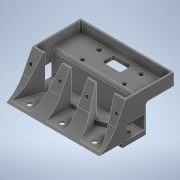
# Autodesk Inventor part: Corpo
Saved by Autodesk Inventor 2021 (Build 250183000, 183)
## iProperties
Created: 2022-11-17
Part Number: Corpo
Material: Plástico PC/ABS
Document SubType Name: Modeling
Designer: nicho
Density: 0.357273 g/cm^3
Appearance: Liso - Preto
Mass: 16.6236 g
Surface Area: 359.302 cm^2
Volume: 46.5292 cm^3
Author: nicho
Autodesk Inventor part; units mm, degrees
ref_plane "YZ Plane" through (0, 0, 0) normal (1, 0, 0) x (0, 1, 0)
ref_plane "XZ Plane" through (0, 0, 0) normal (0, 1, 0) x (-1, 0, 0)
ref_plane "XY Plane" through (0, 0, 0) normal (0, 0, 1) x (1, 0, 0)
sketch "Esboço1" plane through (0, 0, 0) normal (1, 0, 0) x (0, 1, 0)
  line L0 (-19.25, -25) -> (19.25, -25)
  line L1 (19.25, -25) -> (19.25, 25)
  line L2 (19.25, 25) -> (-19.25, 25)
  line L3 (-19.25, 25) -> (-19.25, -25)
  line L4 (-19.25, -25) -> (19.25, 25) construction
  line L5 (19.25, -25) -> (-19.25, 25) construction
  point P0 (0, 0)
  dimension "d0" = 38.5
  dimension "d1" = 50
  constraints: 12 end point, 2 midpoint, 2 parallel, 1 horizontal, 1 perpendicular
  measures "d0" distance of L2.end L1.end
  measures "d1" distance of L1.end L0.end
extrude "Extrusão1" add sketch "Esboço1" along normal mid plane 100
sketch "Esboço2" plane through (50, 0, 0) normal (1, 0, 0) x (0, 0, -1)
  line L0 (25, 19.25) -> (-25, 19.25) projected
  line L1 (25, 19.25) -> (23.5, 19.25)
  line L2 (23.5, 19.25) -> (3, 19.25)
  line L3 (-25, 19.25) -> (-25, -19.25) construction
  line L4 (-25, -19.25) -> (-40.6046, -27.5471) construction
  line L5 (-40.6046, -27.5471) -> (0.8044, -27.5471) construction
  circle A0 centre (-44.3905, 17.2183) radius 41.3029
  line L6 (-7.5894, -1.5328) -> (3, 19.25)
  line L7 (25, 19.25) -> (-25, 19.25) projected
  line L8 (-25, 19.25) -> (-25, -19.25) projected
  line L9 (-25, -19.25) -> (25, -19.25) projected
  line L10 (25, -19.25) -> (25, 19.25) projected
  point P0 (0, 0)
  dimension "d4" = 1.5
  dimension "d5" = 20.5
  dimension "d6" = 28
  dimension "d7" = 63
  constraints: 10 end point, 2 point on circle, 2 point on line, 2 tangent, 1 centre point, 1 perpendicular
  measures "d4" distance of L0.start L1.end
  measures "d5" distance of L1.end L2.end
  measures "d6" angle of L5 L4
  measures "d7" angle of L5 L6
extrude "Extrusão2" cut sketch "Esboço2" against normal through all contours L6 A0 L0 | L8 L0 A0 picked at (-22.6753, -4.8585)
sketch "Esboço3" plane through (-50, 19.25, -25) normal (0, 1, 0) x (1, 0, 0)
  line L0 (0, -22) -> (100, -22) projected
  line L1 (100, 0) -> (100, -22) projected
  line L2 (100, 0) -> (0, 0) projected
  line L3 (0, -22) -> (0, 0) projected
  line L4 (1.5, -1.5) -> (98.5, -1.5)
  line L5 (98.5, -1.5) -> (98.5, -20.5)
  line L6 (98.5, -20.5) -> (1.5, -20.5)
  line L7 (1.5, -20.5) -> (1.5, -1.5)
  point P0 (98.5, -22)
  point P1 (1.5, -22)
  dimension "d14" = 1.5
  constraints: 8 end point, 2 point on line, 3 other
  measures "d14" distance between parallel lines of L2 L4
extrude "Extrusão3" cut sketch "Esboço3" against normal blind 37 contours L4 L5 L6 L7
ref_plane "Plano de trabalho1" through (-48.5, -17.75, -23.5) normal (0, 1, 0) x (1, 0, 0)
sketch "Esboço4" plane through (-48.5, -17.75, -23.5) normal (0, 1, 0) x (1, 0, 0)
  line L0 (39, -19) -> (58, -19)
  line L1 (58, -19) -> (58, -109.0722)
  line L2 (58, -109.0722) -> (39, -109.0722)
  line L3 (39, -109.0722) -> (39, -19)
  line L4 (39, -19) -> (58, -109.0722) construction
  line L5 (58, -19) -> (39, -109.0722) construction
  line L6 (97, -19) -> (0, -19) projected
  line L7 (-1.5, -20.5) -> (-1.5, 1.5) projected
  line L8 (10.7728, -19) -> (28.62, -25.5174)
  line L9 (28.62, -25.5174) -> (-1.8924, -109.0722)
  line L10 (-1.8924, -109.0722) -> (-19.7396, -102.5548)
  line L11 (-19.7396, -102.5548) -> (10.7728, -19)
  line L12 (-1.5, -48.5) -> (98.5, -48.5) projected
  line L13 (-1.5, -48.5) -> (-1.5, -31.0894) projected
  line L14 (48.5, -64.0361) -> (48.5, 0)
  line L15 (0, 0) -> (97, 0) projected
  line L16 (86.2272, -19) -> (68.38, -25.5174)
  line L17 (68.38, -25.5174) -> (98.8924, -109.0722)
  line L18 (98.8924, -109.0722) -> (116.7396, -102.5548)
  line L19 (116.7396, -102.5548) -> (86.2272, -19)
  line L20 (-1.5, -31.0894) -> (-1.5, -20.5) projected
  line L21 (98.5, -31.0894) -> (-1.5, -31.0894) projected
  line L22 (98.5, -20.5) -> (98.5, -31.0894) projected
  line L23 (-1.5, -20.5) -> (98.5, -20.5) projected
  line L24 (-1.5, -48.5) -> (-1.5, -31.0894) projected
  line L25 (-1.5, -48.5) -> (98.5, -48.5) projected
  line L26 (98.5, -31.0894) -> (98.5, -48.5) projected
  line L27 (98.5, -31.0894) -> (-1.5, -31.0894) projected
  line L28 (97, 0) -> (97, -19) projected
  line L29 (97, -19) -> (0, -19) projected
  line L30 (0, -19) -> (0, 0) projected
  line L31 (0, 0) -> (97, 0) projected
  line L32 (-1.5, -20.5) -> (98.5, -20.5) projected
  line L33 (98.5, 1.5) -> (98.5, -20.5) projected
  line L34 (98.5, 1.5) -> (-1.5, 1.5) projected
  line L35 (-1.5, -20.5) -> (-1.5, 1.5) projected
  line L36 (28.62, -25.5174) -> (31, -19)
  line L37 (97, -19) -> (0, -19) projected
  line L38 (68.38, -25.5174) -> (66, -19)
  point P0 (48.5, -23.5)
  point P1 (0, -48.5)
  point P2 (86.2272, -19)
  dimension "d15" = 19
  dimension "d16" = 50
  dimension "d17" = 19
  dimension "d19" = 1.5
  dimension "d90" = 8
  constraints: 34 end point, 5 point on line, 4 parallel, 4 symmetric about line, 3 midpoint, 2 collinear, 2 perpendicular, 1 horizontal, 1 horizontal alignment, 2 other
  measures "d15" distance of L1.end L2.end
  measures "d16" distance from line of L7 L14.start
  measures "d17" distance between parallel lines of L9 L11
  measures "d19" distance from line of L13 point (0, -48.5)
  measures "d90" distance from line of L3 L36.end
extrude "Extrusão4" cut sketch "Esboço4" along normal through all contours L0 L14 L23 L3 | L0 L1 L23 L14 | L23 L14 L21 L3 | L36 L23 L8 L6 | L23 L1 L21 L14 | L21 L14 L12 L3 | L36 L8 L23 | L8 L23 L11 | L6 L16 L23 L38 | L21 L1 L12 L14 | L12 L1 L2 L3 | L21 L11 L23 L8 L9 | L9 L12 L11 L21 | L23 L16 L38 | L19 L23 L16 | L9 L10 L11 L12 | L21 L19 L12 L17 | L17 L16 L23 L19 L21 | L12 L19 L18 L17
sketch "Esboço8" plane through (-50, -19.25, -25) normal (0, -1, 0) x (1, 0, 0)
  line L0 (100, 50) -> (100, 0) projected
  line L1 (0, 0) -> (0, 50) projected
  line L2 (100, 0) -> (0, 0)
  line L3 (0, 0) -> (0, 25)
  line L4 (0, 25) -> (100, 25)
  line L5 (100, 25) -> (100, 0)
  point P0 (50, 25)
  dimension "d32" = 25
  constraints: 8 end point, 2 parallel, 1 horizontal, 1 midpoint, 1 perpendicular
  measures "d32" distance of L2.end L3.end
extrude "Extrusão7" add sketch "Esboço8" along normal blind 4.85
sketch "Esboço10" plane through (-50, -17.75, -25) normal (0, 1, 0) x (1, 0, 0)
  line L0 (40.5, -20.5) -> (32.5, -20.5) projected
  line L1 (12.2728, -20.5) -> (32.5, -20.5)
  line L2 (40.5, -20.5) -> (59.5, -20.5)
  line L3 (67.5, -20.5) -> (59.5, -20.5) projected
  line L4 (98.5, -20.5) -> (87.7272, -20.5) projected
  line L5 (67.5, -20.5) -> (87.7272, -20.5)
  line L6 (7.858, -32.5894) -> (11.725, -22) projected
  line L7 (98.5, -20.5) -> (87.7272, -20.5) projected
  line L8 (98.5, -1.5) -> (98.5, -20.5) projected
  line L9 (1.5, -1.5) -> (98.5, -1.5) projected
  line L10 (1.5, -20.5) -> (1.5, -1.5) projected
  line L11 (12.2728, -20.5) -> (1.5, -20.5) projected
  line L12 (12.2728, -20.5) -> (2.4458, -47.4099) projected
  line L13 (22.6731, -47.4099) -> (2.4458, -47.4099) projected
  line L14 (22.6731, -47.4099) -> (32.5, -20.5) projected
  line L15 (40.5, -20.5) -> (32.5, -20.5) projected
  line L16 (40.5, -20.5) -> (40.5, -47.4099) projected
  line L17 (59.5, -47.4099) -> (40.5, -47.4099) projected
  line L18 (59.5, -47.4099) -> (59.5, -20.5) projected
  line L19 (67.5, -20.5) -> (59.5, -20.5) projected
  line L20 (67.5, -20.5) -> (77.3269, -47.4099) projected
  line L21 (97.5542, -47.4099) -> (77.3269, -47.4099) projected
  line L22 (97.5542, -47.4099) -> (87.7272, -20.5) projected
  line L23 (31.9522, -22) -> (28.0852, -32.5894) projected
  line L24 (88.275, -22) -> (100, -22) projected
  line L25 (0, -25) -> (100, -25) projected
  line L26 (40.5, -20.5) -> (40.5, -47.4099) projected
  line L27 (59.5, -22) -> (59.5, -32.5894) projected
  line L28 (71.9148, -32.5894) -> (68.0478, -22) projected
  line L29 (88.275, -22) -> (92.142, -32.5894) projected
  line L30 (12.2728, -20.5) -> (2.4458, -47.4099) projected
  line L31 (22.6731, -47.4099) -> (32.5, -20.5) projected
  line L32 (31.9522, -22) -> (40.5, -22) projected
  line L33 (40.5, -22) -> (59.5, -22)
  line L34 (69.1433, -25) -> (77.3585, -22)
  line L35 (0, -22) -> (11.725, -22) projected
  line L36 (21.1494, -21.4551) -> (30.8567, -25)
  line L37 (21.1494, -21.4551) -> (21.1494, -20.5)
  line L38 (77.3585, -22) -> (77.3585, -20.5)
  point P0 (50, -25)
  constraints: 16 end point, 7 point on line, 4 horizontal, 4 perpendicular, 1 horizontal alignment
extrude "Extrusão9" add sketch "Esboço10" along normal blind 5 contours L2 L18 L33 L16 | L14 L36 L37 L1 | L5 L38 L34 L20
sketch "Esboço11" plane through (-50, -17.75, -25) normal (0, 1, 0) x (1, 0, 0)
  line L0 (98.5, -20.5) -> (87.7272, -20.5) projected
  line L1 (98.5, -1.5) -> (98.5, -20.5) projected
  line L2 (1.5, -1.5) -> (98.5, -1.5) projected
  line L3 (1.5, -20.5) -> (1.5, -1.5) projected
  line L4 (12.2728, -20.5) -> (1.5, -20.5) projected
  line L5 (12.2728, -20.5) -> (2.4458, -47.4099) projected
  line L6 (22.6731, -47.4099) -> (2.4458, -47.4099) projected
  line L7 (22.6731, -47.4099) -> (30.8567, -25) projected
  line L8 (77.3585, -20.5) -> (21.1494, -20.5) projected
  line L9 (77.3585, -20.5) -> (77.3585, -22) projected
  line L10 (77.3585, -22) -> (69.1433, -25) projected
  line L11 (69.1433, -25) -> (77.3269, -47.4099) projected
  line L12 (97.5542, -47.4099) -> (77.3269, -47.4099) projected
  line L13 (97.5542, -47.4099) -> (87.7272, -20.5) projected
  line L14 (30.8567, -25) -> (21.1494, -21.4551) projected
  line L15 (21.1494, -21.4551) -> (21.1494, -20.5) projected
  line L16 (98.5, -20.5) -> (87.7272, -20.5) projected
  line L17 (12.2728, -20.5) -> (87.7272, -20.5)
  point P0 (50, -25)
  point P1 (21.1494, -20.5)
  constraints: 2 end point, 1 horizontal
extrude "Extrusão10" cut sketch "Esboço11" against normal blind 4.85 contours L0 L17 L8 L4 L3 L2 L1
sketch "Esboço12" plane through (-50, 0, 0) normal (-1, 0, 0) x (0, 0, 1)
  line L0 (-23.5, -19.1) -> (-4.5, -19.1)
  line L1 (-4.5, -19.1) -> (-4.5, -4.1)
  line L2 (-4.5, -4.1) -> (-23.5, -4.1)
  line L3 (-23.5, -4.1) -> (-23.5, -19.1)
  line L4 (-25, 19.25) -> (-25, -24.1) projected
  line L5 (0, -24.1) -> (-25, -24.1) projected
  point P0 (0, 0)
  dimension "d41" = 19
  dimension "d42" = 15
  dimension "d43" = 1.5
  dimension "d44" = 5
  constraints: 8 end point, 2 parallel, 1 horizontal, 1 perpendicular
  measures "d41" distance of L2.end L1.end
  measures "d42" distance of L1.end L0.end
  measures "d43" distance between parallel lines of L4 L3
  measures "d44" distance between parallel lines of L5 L0
extrude "Extrusão11" cut sketch "Esboço12" against normal through all
sketch "Esboço13" plane through (-50, -22.6, -25) normal (0, 1, 0) x (1, 0, 0)
  line L0 (1.5, -1.5) -> (98.5, -1.5) projected
  line L1 (98.5, -20.5) -> (1.5, -20.5) projected
  line L2 (1.5, -1.5) -> (16, -1.5)
  line L3 (16, -1.5) -> (16, -20.5)
  line L4 (16, -20.5) -> (1.5, -20.5)
  line L5 (1.5, -20.5) -> (1.5, -1.5)
  line L6 (98.5, -20.5) -> (98.5, -1.5) projected
  line L7 (59.5, -20.5) -> (67.5, -20.5) projected
  line L8 (98.5, -1.5) -> (84, -1.5)
  line L9 (84, -1.5) -> (84, -20.5)
  line L10 (84, -20.5) -> (98.5, -20.5)
  line L11 (98.5, -20.5) -> (98.5, -1.5)
  point P0 (50, -25)
  point P1 (87.7272, -20.5)
  point P2 (84, -1.5)
  dimension "d47" = 14.5
  dimension "d48" = 14.5
  constraints: 16 end point, 4 parallel, 2 perpendicular, 2 point on line, 1 horizontal
  measures "d47" distance of L3.end L4.end
  measures "d48" distance of L10.end L9.end
extrude "Extrusão12" add sketch "Esboço13" along normal up to surface (3.5 mm away) contours L0 L3 L1 L5 | L0 L6 L1 L9
sketch "Esboço14" plane through (-50, -19.1, -4.5) normal (0, 1, 0) x (1, 0, 0)
  line L0 (16, 19) -> (16, 0) projected
  line L1 (100, 0) -> (0, 0) projected
  line L2 (16, 19) -> (14.5, 19)
  line L3 (14.5, 19) -> (14.5, 0)
  line L4 (14.5, 0) -> (16, 0)
  line L5 (16, 0) -> (16, 19)
  line L6 (84, 19) -> (100, 19) projected
  line L7 (59.5, 0) -> (67.5, 0) projected
  line L8 (84, 19) -> (85.5, 19)
  line L9 (85.5, 19) -> (85.5, 0)
  line L10 (85.5, 0) -> (84, 0)
  line L11 (84, 0) -> (84, 19)
  point P0 (50, -4.5)
  point P1 (87.7272, 0)
  point P2 (84, 0)
  dimension "d51" = 1.5
  dimension "d52" = 1.5
  constraints: 16 end point, 4 parallel, 2 horizontal, 2 perpendicular, 2 point on line
  measures "d51" distance of L4.end L3.end
  measures "d52" distance of L9.end L10.end
extrude "Extrusão13" add sketch "Esboço14" along normal up to surface (6.35 mm away)
sketch "Esboço15" plane through (50, 19.25, -25) normal (0, 0, -1) x (-1, 0, 0)
  line L0 (0, 0) -> (0, -20.7828) projected
  line L1 (100, 0) -> (100, -43.35) projected
  line L2 (0, 0) -> (100, 0)
  line L3 (100, 0) -> (100, -13)
  line L4 (100, -13) -> (0, -13)
  line L5 (0, -13) -> (0, 0)
  point P0 (50, -19.25)
  point P1 (0, -13)
  dimension "d55" = 13
  constraints: 8 end point, 2 parallel, 1 horizontal, 1 perpendicular, 1 point on line
  measures "d55" distance between parallel lines of L2 L4
extrude "Extrusão14" add sketch "Esboço15" along normal blind 30
sketch "Esboço16" plane through (-50, 6.25, -25) normal (0, -1, 0) x (1, 0, 0)
  line L0 (77.5, -30) -> (22.5, -30)
  line L1 (22.5, -30) -> (22.5, 0)
  line L2 (22.5, 0) -> (77.5, 0)
  line L3 (77.5, 0) -> (77.5, -30)
  line L4 (77.5, -30) -> (22.5, 0) construction
  line L5 (22.5, -30) -> (77.5, 0) construction
  line L6 (0, 0) -> (100, 0) projected
  line L7 (100, -30) -> (0, -30) projected
  line L8 (0, 0) -> (0, -30) projected
  point P0 (50, 25)
  point P1 (50, -15)
  dimension "d58" = 55
  dimension "d59" = 50
  constraints: 12 end point, 2 midpoint, 2 parallel, 2 point on line, 1 horizontal, 1 perpendicular
  measures "d58" distance of L1.end L2.end
  measures "d59" distance from line of L8 point (50, -15)
extrude "Extrusão15" add sketch "Esboço16" along normal blind 2.85 contours L0 L1 L2 L3
sketch "Esboço17" plane through (-48.5, 19.25, -23.5) normal (0, 1, 0) x (1, 0, 0)
  line L0 (97, 0) -> (97, -19) projected
  line L1 (97, 0) -> (0, 0)
  line L2 (0, 0) -> (0, 30)
  line L3 (0, 30) -> (97, 30)
  line L4 (97, 30) -> (97, 0)
  line L5 (86.2272, -19) -> (86.775, -20.5) projected
  line L6 (86.775, -20.5) -> (98.5, -20.5) projected
  line L7 (98.5, -20.5) -> (98.5, 31.5) projected
  line L8 (-1.5, 31.5) -> (98.5, 31.5) projected
  line L9 (-1.5, -20.5) -> (-1.5, 31.5) projected
  line L10 (-1.5, -20.5) -> (10.225, -20.5) projected
  line L11 (10.225, -20.5) -> (10.7728, -19) projected
  line L12 (10.7728, -19) -> (0, -19) projected
  line L13 (0, -19) -> (0, 0) projected
  line L14 (0, 0) -> (97, 0) projected
  line L15 (97, 0) -> (97, -19) projected
  line L16 (97, -19) -> (86.2272, -19) projected
  point P0 (48.5, -23.5)
  dimension "d62" = 1.5
  constraints: 8 end point, 2 parallel, 1 horizontal, 1 perpendicular, 1 point on line
  measures "d62" distance between parallel lines of L8 L3
extrude "Extrusão16" cut sketch "Esboço17" against normal blind 11.5 contours L1 L2 L3 L4
fillet "Arredondamento2" radius 2.85 3 edges at (0, 7.75, -23.5) (38.75, 6.25, -25) (-38.75, 6.25, -25)
fillet "Arredondamento3" radius 1.5 4 edges at (-48.5, 13.5, -53.5) (48.5, 13.5, -53.5) (48.5, 7.575, -4.5) (-48.5, 7.575, -4.5)
sketch "Esboço18" plane through (-50, 3.4, -25) normal (0, -1, 0) x (1, 0, 0)
  line L0 (0, 0) -> (100, 0) projected
  line L1 (77.5, -30) -> (77.5, 0) projected
  line L2 (22.5, 0) -> (22.5, -30) projected
  line L3 (22.5, -30) -> (77.5, -30) projected
  point P0 (50, 25)
  point P1 (72.5, -22.5)
  point P2 (27.5, -22.5)
  point P3 (27.5, -4.5)
  point P4 (72.5, -4.5)
  dimension "d69" = 4.5
  dimension "d70" = 5
  dimension "d71" = 5
  dimension "d72" = 7.5
  constraints: 2 horizontal alignment, 2 vertical alignment
  measures "d69" distance from line of L0 point (72.5, -4.5)
  measures "d70" distance from line of L1 point (72.5, -4.5)
  measures "d71" distance from line of L2 point (27.5, -4.5)
  measures "d72" distance from line of L3 point (72.5, -22.5)
hole "Furo1" at (22.5, 3.4, -47.5) at (-22.5, 3.4, -47.5) at (-22.5, 3.4, -29.5) at (22.5, 3.4, -29.5) direction (0, 1, 0) diameter 4 end through all start extended yes
chamfer "Chanfro1" distance 1 angle 45 4 edges at (-22.5, 7.75, -45.5) (-22.5, 7.75, -27.5) (22.5, 7.75, -27.5) (22.5, 7.75, -45.5)
sketch "Esboço19" plane through (-48.5, 7.75, -23.5) normal (0, 1, 0) x (1, 0, 0)
  line L0 (38.5, 26.5) -> (58.5, 26.5)
  line L1 (58.5, 26.5) -> (58.5, 14)
  line L2 (58.5, 14) -> (38.5, 14)
  line L3 (38.5, 14) -> (38.5, 26.5)
  line L4 (38.5, 26.5) -> (58.5, 14) construction
  line L5 (58.5, 26.5) -> (38.5, 14) construction
  line L6 (-1.5, -20.5) -> (-1.5, 31.5) projected
  line L7 (-1.5, 31.5) -> (98.5, 31.5) projected
  point P0 (48.5, -23.5)
  point P1 (48.5, 20.25)
  dimension "d83" = 20
  dimension "d84" = 12.5
  dimension "d85" = 50
  dimension "d86" = 5
  constraints: 12 end point, 2 midpoint, 2 parallel, 1 horizontal, 1 perpendicular
  measures "d83" distance of L1.end L2.end
  measures "d84" distance of L0.end L1.end
  measures "d85" distance from line of L6 point (48.5, 20.25)
  measures "d86" distance between parallel lines of L7 L0
extrude "Extrusão17" cut sketch "Esboço19" against normal through all
fillet "Arredondamento5" radius 2 4 edges at (-10, 5.575, -37.5) (10, 5.575, -37.5) (-10, 5.575, -50) (10, 5.575, -50)
sketch "Esboço20" plane through (-50, -17.75, -25) normal (0, 1, 0) x (1, 0, 0)
  line L0 (0, -22) -> (0, 30) projected
  line L1 (0, -50) -> (100, -50) projected
  line L2 (2.4458, -47.4099) -> (7.858, -32.5894) projected
  line L3 (92.142, -32.5894) -> (97.5542, -47.4099) projected
  point P0 (50, -25)
  point P1 (50, -40)
  point P2 (15, -40)
  point P3 (85, -40)
  dimension "d91" = 50
  dimension "d92" = 10
  dimension "d120" = 35
  dimension "d121" = 35
  constraints: 2 horizontal alignment
  measures "d91" distance from line of L0 point (50, -40)
  measures "d92" distance from line of L1 point (50, -40)
  measures "d120" distance of point (15, -40) point (50, -40)
  measures "d121" distance of point (85, -40) point (50, -40)
hole "Furo2" at (0, -17.75, 15) at (-35, -17.75, 15) at (35, -17.75, 15) direction (0, -1, 0) diameter 4 end through all start extended yes countersink diameter 6 countersink angle 90
sketch "Esboço21" plane through (-50, -19.1, -4.5) normal (0, 1, 0) x (1, 0, 0)
  line L0 (0, -1.5) -> (0, 50.5) projected
  line L1 (100, -1.5) -> (100, 50.5) projected
  line L2 (12.2728, 0) -> (3, 0) projected
  circle A0 centre (50, -19.5) radius 2 projected
  point P0 (50, -4.5)
  point P1 (7, 9.5)
  point P2 (93, 9.5)
  dimension "d126" = 29
  dimension "d127" = 43
  dimension "d128" = 43
  constraints: 1 horizontal alignment
  measures "d126" vertical distance of A0.centre point (7, 9.5)
  measures "d127" horizontal distance of A0.centre point (7, 9.5)
  measures "d128" horizontal distance of point (93, 9.5) A0.centre
hole "Furo3" at (-43, -19.1, -14) at (43, -19.1, -14) direction (0, -1, 0) diameter 4 end through all start extended yes countersink diameter 6 countersink angle 90
sketch "Esboço22" plane through (-50, -22.6, -25) normal (0, 1, 0) x (1, 0, 0)
  circle A0 centre (7, -11) radius 3 projected
  line L0 (14.5, -20.5) -> (14.5, -1.5) projected
  line L1 (0, -1.5) -> (14.5, -1.5) projected
  line L2 (0, -20.5) -> (0, -1.5) projected
  line L3 (14.5, -20.5) -> (0, -20.5) projected
  circle A1 centre (50, -40) radius 3 projected
  line L4 (59.5, -25) -> (40.5, -25) projected
  line L5 (40.5, -25) -> (40.5, -47.4099) projected
  line L6 (59.5, -47.4099) -> (40.5, -47.4099) projected
  line L7 (59.5, -47.4099) -> (59.5, -25) projected
  line L8 (85.5, -1.5) -> (85.5, -20.5) projected
  line L9 (100, -1.5) -> (100, -20.5) projected
  line L10 (85.5, -1.5) -> (100, -1.5) projected
  line L11 (100, -20.5) -> (85.5, -20.5) projected
  point P0 (50, -25)
  point P1 (50, -11)
  constraints: 1 horizontal alignment, 1 vertical alignment
hole "Furo4" at (0, -22.6, -14) direction (0, -1, 0) diameter 4 end through all start extended yes countersink diameter 6 countersink angle 90
ref_plane "Plano de trabalho2" through (-9.5, 19.25, -3) normal (0, 0.4539905, 0.8910065) x (1, 0, 0)
sketch "Esboço23" plane through (-9.5, 19.25, -3) normal (0, 0.4539905, 0.8910065) x (1, 0, 0)
  line L0 (0, -23.3251) -> (0, 0) projected
  line L1 (-8.5478, 0) -> (0, 0) projected
  line L2 (-8.5478, 0) -> (-12.4148, -23.3251) projected
  line L3 (0, -23.3251) -> (-12.4148, -23.3251) projected
  line L4 (31.4148, -23.3251) -> (27.5478, 0) projected
  line L5 (19, 0) -> (27.5478, 0) projected
  line L6 (19, 0) -> (19, -23.3251) projected
  line L7 (31.4148, -23.3251) -> (19, -23.3251) projected
  line L8 (47.775, 0) -> (51.642, -23.3251) projected
  line L9 (59.5, -23.3251) -> (51.642, -23.3251) projected
  line L10 (59.5, 0) -> (59.5, -23.3251) projected
  line L11 (47.775, 0) -> (59.5, 0) projected
  line L12 (-32.642, -23.3251) -> (-28.775, 0) projected
  line L13 (-40.5, 0) -> (-28.775, 0) projected
  line L14 (-40.5, -23.3251) -> (-40.5, 0) projected
  line L15 (-32.642, -23.3251) -> (-40.5, -23.3251) projected
  point P0 (9.5, -18.5138)
  point P1 (-5, -13.3251)
  point P2 (-36.5, -13.3251)
  point P3 (24, -13.3251)
  point P4 (55.5, -13.3251)
  dimension "d129" = 4
  dimension "d130" = 4
  dimension "d131" = 5
  dimension "d132" = 5
  dimension "d133" = 10
  constraints: 3 horizontal alignment
  measures "d129" distance from line of L10 point (55.5, -13.325)
  measures "d130" distance from line of L14 point (-36.5, -13.325)
  measures "d131" distance from line of L0 point (-5, -13.325)
  measures "d132" distance from line of L6 point (24, -13.325)
  measures "d133" distance from line of L7 point (24, -13.325)
hole "Furo5" at (-14.5, 7.3772, 3.0495) at (-46, 7.3772, 3.0495) at (14.5, 7.3772, 3.0495) at (46, 7.3772, 3.0495) direction (0, -0.4539905, -0.8910065) diameter 4 depth 5 start extended yes
sketch "Esboço24" plane through (-50, -17.75, -25) normal (0, 1, 0) x (1, 0, 0)
  circle A0 centre (15, -40) radius 3 projected
  line L0 (87.7272, -20.5) -> (85.5, -20.5) projected
  line L1 (16, -20.5) -> (14.5, -20.5) projected
  line L2 (14.5, -20.5) -> (12.2728, -20.5) projected
  line L3 (12.2728, -20.5) -> (2.4458, -47.4099) projected
  line L4 (22.6731, -47.4099) -> (2.4458, -47.4099) projected
  line L5 (22.6731, -47.4099) -> (30.8567, -25) projected
  line L6 (30.8567, -25) -> (21.1494, -21.4551) projected
  line L7 (21.1494, -21.4551) -> (21.1494, -20.5) projected
  circle A1 centre (85, -40) radius 3 projected
  line L8 (87.7272, -20.5) -> (85.5, -20.5) projected
  line L9 (85.5, -20.5) -> (84, -20.5) projected
  line L10 (84, -20.5) -> (77.3585, -20.5) projected
  line L11 (77.3585, -20.5) -> (77.3585, -22) projected
  line L12 (77.3585, -22) -> (69.1433, -25) projected
  line L13 (69.1433, -25) -> (77.3269, -47.4099) projected
  line L14 (97.5542, -47.4099) -> (77.3269, -47.4099) projected
  line L15 (97.5542, -47.4099) -> (87.7272, -20.5) projected
  line L16 (21.1494, -21.4551) -> (30.8567, -25) projected
  line L17 (21.1494, -21.4551) -> (16, -19.5747)
  line L18 (77.3585, -22) -> (84, -19.5747)
  line L19 (69.1433, -25) -> (77.3585, -22) projected
  line L20 (32.5, -20.5) -> (21.1494, -20.5) projected
  line L21 (21.1494, -20.5) -> (16, -18.6196)
  line L22 (16, -1.5) -> (16, -20.5) projected
  line L23 (77.3585, -22) -> (77.3585, -20.5) projected
  line L24 (77.3585, -20.5) -> (84, -18.0747)
  line L25 (84, -20.5) -> (84, -1.5) projected
  line L26 (21.1494, -20.5) -> (16, -20.5) projected
  line L27 (16, -20.5) -> (14.5, -20.5) projected
  line L28 (14.5, -20.5) -> (12.2728, -20.5) projected
  line L29 (12.2728, -20.5) -> (2.4458, -47.4099) projected
  line L30 (22.6731, -47.4099) -> (2.4458, -47.4099) projected
  line L31 (22.6731, -47.4099) -> (30.8567, -25) projected
  line L32 (30.8567, -25) -> (21.1494, -21.4551) projected
  line L33 (21.1494, -21.4551) -> (21.1494, -20.5) projected
  line L34 (85.5, -20.5) -> (84, -20.5) projected
  line L35 (84, -20.5) -> (77.3585, -20.5) projected
  line L36 (77.3585, -20.5) -> (77.3585, -22) projected
  line L37 (77.3585, -22) -> (69.1433, -25) projected
  line L38 (69.1433, -25) -> (77.3269, -47.4099) projected
  line L39 (97.5542, -47.4099) -> (77.3269, -47.4099) projected
  line L40 (97.5542, -47.4099) -> (87.7272, -20.5) projected
  line L41 (21.1494, -20.5) -> (16, -20.5) projected
  point P0 (50, -25)
  point P1 (16, -17.5)
  point P2 (84, -17.5)
  point P3 (16, -4.5)
  point P4 (84, -4.5)
  point P5 (81.466, -20.5)
  point P6 (18.534, -20.5)
  constraints: 8 end point, 2 collinear, 2 parallel, 2 point on line
extrude "Extrusão18" add sketch "Esboço24" along normal mid plane 10 contours L10 L18 L25 | L18 L11 L10 | L10 L24 L25 L18 | L22 L17 L26 | L22 L21 L26 L17 | L26 L7 L17
sketch "Esboço26" plane through (-50, -12.75, -25) normal (0, 1, 0) x (1, 0, 0)
  line L0 (18.534, -20.5) -> (30.8567, -25) projected
  line L1 (18.534, -20.5) -> (14.5, -19.0269)
  line L2 (14.5, -20.5) -> (14.5, -1.5) projected
  line L3 (21.1494, -20.5) -> (16, -18.6196) projected
  line L4 (18.534, -20.5) -> (30.8567, -25) projected
  line L5 (32.5, -20.5) -> (30.8567, -25) projected
  line L6 (32.5, -20.5) -> (21.1494, -20.5) projected
  line L7 (21.1494, -20.5) -> (16, -18.6196) projected
  line L8 (16, -1.5) -> (16, -18.6196) projected
  line L9 (14.5, -1.5) -> (16, -1.5) projected
  line L10 (14.5, -20.5) -> (14.5, -1.5) projected
  line L11 (14.5, -20.5) -> (18.534, -20.5) projected
  line L12 (85.5, -20.5) -> (81.466, -20.5) projected
  line L13 (85.5, -1.5) -> (85.5, -20.5) projected
  line L14 (84, -1.5) -> (85.5, -1.5) projected
  line L15 (84, -18.0747) -> (84, -1.5) projected
  line L16 (84, -18.0747) -> (77.3585, -20.5) projected
  line L17 (77.3585, -20.5) -> (67.5, -20.5) projected
  line L18 (69.1433, -25) -> (67.5, -20.5) projected
  line L19 (69.1433, -25) -> (81.466, -20.5) projected
  line L20 (85.5, -20.5) -> (81.466, -20.5) projected
  line L21 (81.466, -20.5) -> (85.5, -19.0269)
  line L22 (84, -18.0747) -> (77.3585, -20.5) projected
  point P0 (50, -25)
  constraints: 4 end point, 2 parallel, 2 point on line
extrude "Extrusão19" cut sketch "Esboço26" against normal up to surface (5 mm away) contours L11 L2 L1 | L12 L21 L13
fillet "Arredondamento6" radius 4 6 edges at (34, -17.675, -23.5) (-34, -17.675, -23.5) (-34, -17.675, -6.3804) (-28.8506, -17.675, -4.5) (34, -17.675, -6.9253) (27.3585, -17.675, -4.5)
sketch "Esboço27" plane through (-50, -19.1, -4.5) normal (0, 1, 0) x (1, 0, 0)
  line L0 (14.5, 0) -> (0, 0) projected
  line L1 (13.25, 0) -> (13.25, 19)
  line L2 (14.5, 1.4731) -> (14.5, 19) projected
  line L3 (14.5, 1.4731) -> (13.25, 1.9296)
  line L4 (14.5, 1.4731) -> (30.8567, -4.5) projected
  line L5 (100, 0) -> (85.5, 0) projected
  line L6 (86.75, 0) -> (86.75, 19)
  line L7 (85.5, 19) -> (85.5, 1.4731) projected
  line L8 (85.5, 1.4731) -> (86.75, 1.9296)
  line L9 (69.1433, -4.5) -> (85.5, 1.4731) projected
  line L10 (1.5, 19) -> (98.5, 19) projected
  point P0 (50, -4.5)
  dimension "d146" = 1.25
  dimension "d147" = 1.25
  constraints: 8 end point, 6 point on line, 2 collinear, 2 vertical
  measures "d146" distance between parallel lines of L2 L1
  measures "d147" distance between parallel lines of L7 L6
extrude "Extrusão20" add sketch "Esboço27" along normal up to surface (6.35 mm away)
fillet "Arredondamento7" radius 1.5 4 edges at (35.5, -18.425, -4.5) (-35.5, -18.425, -4.5) (-36.75, -15.925, -6.4296) (36.75, -15.925, -6.4296)
equation "\"d71\" = d70"
equation "\"d128\" = d127"
